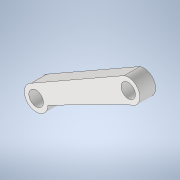
# Autodesk Inventor part: palanca_proxima_media
Saved by Autodesk Inventor 2020.4 (Build 244396010, 396A)
## iProperties
Created: 2021-11-11
Part Number: palanca_proxima_media
Material: Generic
Document SubType Name: Modeling
Designer: chalo
Density: 1 g/cm^3
Appearance: Default
Author: chalo
Autodesk Inventor part; units mm, degrees
ref_plane "YZ Plane" through (0, 0, 0) normal (1, 0, 0) x (0, 1, 0)
ref_plane "XZ Plane" through (0, 0, 0) normal (0, 1, 0) x (-1, 0, 0)
ref_plane "XY Plane" through (0, 0, 0) normal (0, 0, 1) x (1, 0, 0)
sketch "Sketch1" plane through (0, 0, 0) normal (0, 0, 1) x (1, 0, 0)
  circle A0 centre (49.25, 5.6396) radius 1.625 projected
  circle A1 centre (69.7498, 17.4021) radius 1.6 projected
  circle A2 centre (49.25, 5.6396) radius 2.625
  circle A3 centre (69.7498, 17.4021) radius 2.6
  line L0 (50.4505, 7.9739) -> (67.3082, 18.2959)
  line L1 (51.875, 5.6396) -> (68.5894, 15.0754)
  point P0 (0, 0)
  dimension "d0" = 1
  dimension "d1" = 1
  constraints: 4 end point, 4 point on circle, 2 centre point
  measures "d0" radial gap between concentric circles of A0 A2
  measures "d1" radial gap between concentric circles of A1 A3
extrude "Extrusion1" add sketch "Sketch1" along normal mid plane 3.5
body "Solid1"
